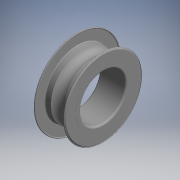
# Autodesk Inventor part: SKF_7205 BE-2RZP_PART1
Saved by Autodesk Inventor 2017.3 (Build 213256000, 256)
## iProperties
Part Number: SKF_7205 BE-2RZP_PART1
Material: Generic
Catalog Web Link: www.cadenas.de
Description: -Angular contact ball bearings, single row
Vendor: SKF
Document SubType Name: Modeling
Designer: partserver
Manufacturer: SKF
Mass: 130 g
Surface Area: 66.8761 cm^2
Volume: 5.78549 cm^3
Density: 1 g/cm^3
Appearance: PSOLRGB-175-175-175
Category: PARTsolutions
Company: SKF
Title: SKF_7205 BE-2RZP_PART1
Author: Cadenas PARTsolutions
Comments: Angular contact ball bearings, single row
PSOL_IDENT_0: {$CADENAS_DATA\23d-libs\skf\bearings_units_and_housings\ball_bearings\angular_contact_ball_bearings\
PSOL_IDENT_1: ba1_001_101.prj},212 {VTYP=3D},{NB=SKF_7205 BE-2RZP_PART1},{LINA=SKF_7205 BE-2RZP_PART1},{NN=BA1_001
PSOL_IDENT_2: _101_PART1},{NOPRJ=TRUE},{DATE=13.09.2021 11:18:32},{GEOMDATE=07.09.2021 05:50:45},{VERSION=},{LINEI
PSOL_IDENT_3: D=141990},{WBVAR=},{WBNUMERIC=}  {NB=SKF_7205 BE-2RZP_PART1},{LINA=SKF_7205 BE-2RZP_PART1},{KT=DUMMY
PSOL_IDENT_4: },{DESIGNATION=7205 BE-2RZP},{DD=25.000},{D=52.000},{B=15.0000},{DD1=35.850},{DD2=30.870},{D1=41.570
PSOL_IDENT_5: },{D2=42.700},{D3=MIN},{D4=46.270},{D5=46.8},{C1=MIN},{AA=24},{R12=1.000},{R34=0.600},{ALPHA=40},{PI
PSOL_IDENT_6: TCH=38.500},{DW=7.938},{DDAMIN=30.6},{DDAMAX=35.5},{DAMAX=46.4},{DBMAX=47.8},{RAMAX=1},{RBMAX=0.6},{
PSOL_IDENT_7: LOAD1=14.8},{LOAD2=9.3},{LOAD3=0.4},{SPEED1=16000},{SPEED2=12000},{Z=13},{II=1},{MASS=0.13},{BEARING=
PSOL_IDENT_8: 7205 BE-2RZP},{POPULAR=Yes},{VARIANT=design_ba1_001_101_1},{D2A=42.7},{DD2A=30.870},{R5R=0.6},{R34L=
PSOL_IDENT_9: 1},{IRH=1},{ORH=1},{D4H=1}
NB: SKF_7205 BE-2RZP_PART1
NT: Angular contact ball bearings, single row
NBSYN: SKF_$DESIGNATION._PART1
LINA: SKF_7205 BE-2RZP_PART1
CATALOG: SKF
DESIGNATION: 7205 BE-2RZP
DD: 25
D: 52
B: 15
LOAD1: 14.8
LOAD2: 9.3
LOAD3: 0.4
SPEED1: 16000
SPEED2: 12000
BEARING: 7205 BE-2RZP
SUPPLIER: SKF
ARTICLENO: SKF_7205 BE-2RZP_PART1
BOMINFO: SKF_7205 BE-2RZP_PART1
CREATOR: CADENAS GmbH
Autodesk Inventor part; units mm, degrees
ref_plane "YZ Plane" through (0, 0, 0) normal (1, 0, 0) x (0, 1, 0)
ref_plane "XZ Plane" through (0, 0, 0) normal (0, 1, 0) x (-1, 0, 0)
ref_plane "XY Plane" through (0, 0, 0) normal (0, 0, 1) x (1, 0, 0)
sketch "Sketch_4" plane through (0, 0, 0) normal (0, 0, 1) x (1, 0, 0)
  line L0 (15, 0) -> (0, 0)
  line L1 (0, 15.435) -> (0, 13.5)
  arc A0 (0, 13.5) -> (1, 12.5) centre (1, 13.5) ccw
  line L2 (1, 12.5) -> (14, 12.5)
  arc A1 (14, 12.5) -> (15, 13.5) centre (14, 13.5) ccw
  line L3 (15, 13.5) -> (15, 17.925)
  line L4 (15, 17.925) -> (11.2413, 17.925)
  arc A2 (6.4051, 15.435) -> (11.2413, 17.925) centre (7.5, 19.25) ccw
  line L5 (6.4051, 15.435) -> (0, 15.435)
  constraints: 12 end point, 6 point on circle, 3 centre point
revolve "Revolution1" add sketch "Sketch_4" angle 360 about axis through (15, 0, 0) along (1, 0, 0)
sketch "Sketch_5" plane through (0, 0, 0) normal (0, 0, 1) x (1, 0, 0)
  line L0 (5, 0) -> (-5, 0)
  line L1 (0.0667, 20.885) -> (0.0667, 15.435)
  line L2 (0.0667, 15.435) -> (0.8333, 15.435)
  line L3 (0.8333, 15.435) -> (0.5667, 15.7017)
  line L4 (0.5667, 15.7017) -> (0.5667, 21.0234)
  arc A0 (0.5667, 21.0234) -> (0.1667, 21.35) centre (0.5, 21.35) ccw
  line L5 (0.1667, 21.35) -> (0.3391, 21.35)
  arc A1 (0.3903, 21.2323) -> (0.3391, 21.35) centre (0.3391, 21.28) ccw
  line L6 (0.3903, 21.2323) -> (0.0667, 20.885)
  constraints: 14 end point, 4 point on circle, 2 centre point
revolve "Revolution2" add sketch "Sketch_5" angle 360 about axis through (5, 0, 0) along (1, 0, 0)
sketch "Sketch_6" plane through (0, 0, 0) normal (0, 0, 1) x (1, 0, 0)
  line L0 (5, 0) -> (-5, 0)
  arc A0 (14.8333, 23.675) -> (14.4333, 23.3484) centre (14.5, 23.675) ccw
  line L1 (14.4333, 23.3484) -> (14.4333, 18.1917)
  line L2 (14.4333, 18.1917) -> (14.1667, 17.925)
  line L3 (14.1667, 17.925) -> (14.9333, 17.925)
  line L4 (14.9333, 17.925) -> (14.9333, 23.375)
  line L5 (14.9333, 23.375) -> (14.7106, 23.5292)
  arc A1 (14.7561, 23.675) -> (14.7106, 23.5292) centre (14.7561, 23.595) ccw
  line L6 (14.7561, 23.675) -> (14.8333, 23.675)
  constraints: 14 end point, 4 point on circle, 2 centre point
revolve "Revolution3" add sketch "Sketch_6" angle 360 about axis through (5, 0, 0) along (1, 0, 0)
body "Solid1"
